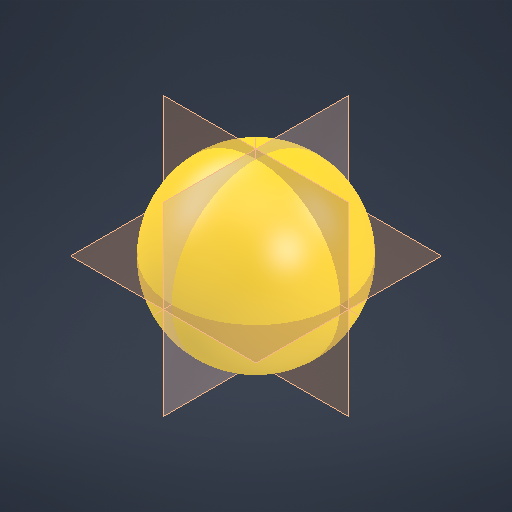
# Autodesk Inventor part: 70mm ball
Saved by Autodesk Inventor 2026.1 (Build 301233020, 233B)
## iProperties
Created: 2025-10-13
Part Number: 70mm ball
Material: Generic
Document SubType Name: Modeling
Designer: User
Density: 1 g/cm^3
Appearance: Default
Author: User
Autodesk Inventor part; units mm, degrees
sketch "Sketch1" plane through (0, 0, 0) normal (0, 1, 0) x (-1, 0, 0)
  arc A0 (0, 35) -> (0, -35) centre (0, 0) ccw
  line L0 (0, -35) -> (0, 35)
  line L1 (0, -49) -> (0, 49) projected
  constraints: 2 end point, 2 point on circle, 1 centre point, 1 coincident, 1 vertical
revolve "Revolution1" add sketch "Sketch1" angle 360 about axis through (0, 0, -10) along (0, 0, 1)
body "Solid1"
